Autodesk Inventor part; units mm, degrees
(part 2 of 2)
sketch "Sketch20" plane through (-59.7998, 7.69, 3.5001) normal (0, 0, -1) x (-1, 0, 0)
  line L0 (4.2162, -20.29) -> (4.2162, 0) construction
  line L1 (4.2162, -21.29) -> (44.8074, -21.29) construction
  line L2 (4.2162, 0) -> (4.2162, -21.29) construction
  line L3 (39.8922, -3) -> (33.5483, -3) construction
  line L4 (39.8922, -3) -> (4.2162, -3) construction
  line L5 (4.2162, -3) -> (4.2162, -21.29) construction
  line L6 (4.2162, -21.29) -> (39.8922, -21.29) construction
  line L7 (39.8922, -21.29) -> (39.8922, -3) construction
  line L8 (4.2162, -3) -> (44.8074, -3) construction
  line L9 (44.8074, -3) -> (44.8074, -21.29) construction
  line L10 (44.8074, -21.29) -> (4.2162, -21.29) construction
  line L11 (4.2162, -21.29) -> (4.2162, -3) construction
  line L12 (44.8074, -12.145) -> (4.2162, -12.145) construction
  circle A0 centre (24.5118, -12.145) radius 3.5
  point P0 (-59.7998, -7.69)
  dimension "d266" = 7
  constraints: 22 end point, 4 parallel, 3 horizontal, 3 midpoint, 2 perpendicular, 1 centre point
  measures "d266" diameter of A0
extrude "Extrusion15" cut sketch "Sketch20" along normal blind 100 and the other way blind 50
sketch "Sketch21" plane through (-66.1, 7.69, -7.6) normal (0, 1, 0) x (1, 0, 0)
  line L0 (71.1002, -14.1001) -> (71.1002, 52.1999) projected
  arc A0 (71.1002, 52.1999) -> (67.2926, 61.3923) centre (58.1002, 52.1999) ccw projected
  line L1 (67.2926, 61.3923) -> (47.1426, 81.5423) projected
  arc A1 (47.1426, 81.5423) -> (28.7578, 81.5423) centre (37.9502, 72.3499) ccw projected
  line L2 (28.7578, 81.5423) -> (8.6078, 61.3923) projected
  arc A2 (8.6078, 61.3923) -> (5.0308, 54.6374) centre (17.8002, 52.1999) ccw projected
  arc A3 (2.084, 52.1999) -> (5.0308, 54.6374) centre (2.084, 55.1999) ccw projected
  line L3 (2.084, 52.1999) -> (-68.9958, 52.1999) projected
  arc A4 (-68.9958, 52.1999) -> (-78.1882, 48.3923) centre (-68.9958, 39.1999) ccw projected
  line L4 (-78.1882, 48.3923) -> (-98.3382, 28.2423) projected
  arc A5 (-98.3382, 28.2423) -> (-98.3382, 9.8575) centre (-89.1458, 19.0499) ccw projected
  line L5 (-98.3382, 9.8575) -> (-78.1882, -10.2925) projected
  arc A6 (-78.1882, -10.2925) -> (-68.9958, -14.1001) centre (-68.9958, -1.1001) ccw projected
  line L6 (-68.9958, -14.1001) -> (2.084, -14.1001) projected
  arc A7 (5.0308, -16.5376) -> (2.084, -14.1001) centre (2.084, -17.1001) ccw projected
  arc A8 (5.0308, -16.5376) -> (8.6078, -23.2925) centre (17.8002, -14.1001) ccw projected
  line L7 (8.6078, -23.2925) -> (28.7578, -43.4425) projected
  arc A9 (28.7578, -43.4425) -> (47.1426, -43.4425) centre (37.9502, -34.2501) ccw projected
  line L8 (47.1426, -43.4425) -> (67.2926, -23.2925) projected
  arc A10 (67.2926, -23.2925) -> (71.1002, -14.1001) centre (58.1002, -14.1001) ccw projected
  line L9 (68.1002, 49.1999) -> (68.1002, -10.3919) projected
  line L10 (68.1002, -10.3919) -> (66.5817, -14.6605) projected
  arc A11 (64.1106, -20.1105) -> (66.5817, -14.6605) centre (58.1002, -14.1001) ccw projected
  line L11 (64.1106, -20.1105) -> (43.9606, -40.2605) projected
  arc A12 (31.9398, -40.2605) -> (43.9606, -40.2605) centre (37.9502, -34.2501) ccw projected
  line L12 (31.9398, -40.2605) -> (11.7898, -20.1105) projected
  arc A13 (9.3002, -14.1001) -> (11.7898, -20.1105) centre (17.8002, -14.1001) ccw projected
  arc A14 (9.3002, -14.1001) -> (6.3002, -11.1001) centre (6.3002, -14.1001) ccw projected
  line L13 (6.3002, -11.1001) -> (-38.5071, -11.1001) projected
  arc A15 (-40.6284, -10.2214) -> (-38.5071, -11.1001) centre (-38.5071, -8.1001) ccw projected
  line L14 (-40.6284, -10.2214) -> (-40.3711, -10.4788) projected
  arc A16 (-40.3711, -10.4788) -> (-42.4924, -9.6001) centre (-42.4924, -12.6001) ccw projected
  line L15 (-42.4924, -9.6001) -> (-68.9958, -9.6001) projected
  arc A17 (-75.0062, -7.1105) -> (-68.9958, -9.6001) centre (-68.9958, -1.1001) ccw projected
  line L16 (-75.0062, -7.1105) -> (-95.1562, 13.0395) projected
  arc A18 (-95.1562, 25.0603) -> (-95.1562, 13.0395) centre (-89.1458, 19.0499) ccw projected
  line L17 (-95.1562, 25.0603) -> (-75.0062, 45.2103) projected
  arc A19 (-68.9958, 47.6999) -> (-75.0062, 45.2103) centre (-68.9958, 39.1999) ccw projected
  line L18 (-68.9958, 47.6999) -> (-42.4924, 47.6999) projected
  arc A20 (-42.4924, 47.6999) -> (-40.3711, 48.5786) centre (-42.4924, 50.6999) ccw projected
  line L19 (-40.3711, 48.5786) -> (-40.3356, 48.6141) projected
  arc A21 (-38.9213, 49.1999) -> (-40.3356, 48.6141) centre (-38.9213, 47.1999) ccw projected
  line L20 (-38.9213, 49.1999) -> (6.3002, 49.1999) projected
  arc A22 (6.3002, 49.1999) -> (9.3002, 52.1999) centre (6.3002, 52.1999) ccw projected
  arc A23 (11.7898, 58.2103) -> (9.3002, 52.1999) centre (17.8002, 52.1999) ccw projected
  line L21 (11.7898, 58.2103) -> (31.9398, 78.3603) projected
  arc A24 (43.9606, 78.3603) -> (31.9398, 78.3603) centre (37.9502, 72.3499) ccw projected
  line L22 (43.9606, 78.3603) -> (64.1106, 58.2103) projected
  arc A25 (66.8919, 51.6165) -> (64.1106, 58.2103) centre (57.0713, 51.3576) ccw projected
  line L23 (66.8919, 51.6165) -> (68.1002, 49.1999) projected
  point P0 (66.1, -7.6)
extrude "Extrusion16" add sketch "Sketch21" against normal blind 3 contours A10 L8 A9 L7 A8 A7 L6 A6 L5 A5 L4 A4 L3 A3 A2 L2 A1 L1 A0 L0 | L9 L10 A11 L11 A12 L12 A13 A14 L13 A15 L14 A16 L15 A17 L16 A18 L17 A19 L18 A20 L19 A21 L20 A22 A23 L21 A24 L22 A25 L23
sketch "Sketch22" plane through (-57.4922, -13.6, 15.6925) normal (-0.7071068, 0, 0.7071068) x (0.7071068, 0, 0.7071068)
  line L0 (44.1622, -18.29) -> (71.0798, -18.29) construction
  line L1 (71.0798, -18.29) -> (71.0798, -1) construction
  line L2 (71.0798, -1) -> (44.1622, -1) construction
  line L3 (44.1622, -1) -> (44.1622, -18.29) construction
  line L4 (71.0798, -1) -> (71.0798, -18.29) construction
  line L5 (71.0798, -9.645) -> (44.1622, -9.645) construction
  line L6 (44.1622, -1) -> (44.1622, -18.29) construction
  arc A0 (55.5252, -6.11) -> (61.6635, -6.11) centre (58.5944, -10) ccw
  line L7 (55.5252, -6.11) -> (61.6635, -6.11)
  line L8 (50.344, -9.645) -> (54.4692, -2.5) construction
  line L9 (54.4692, -2.5) -> (62.7195, -2.5) construction
  line L10 (62.7195, -2.5) -> (66.8447, -9.645) construction
  line L11 (66.8447, -9.645) -> (62.7195, -16.79) construction
  line L12 (62.7195, -16.79) -> (54.4692, -16.79) construction
  line L13 (54.4692, -16.79) -> (50.344, -9.645) construction
  line L14 (58.5944, -9.645) -> (54.4692, -2.5) construction
  line L15 (58.5944, -10) -> (58.5944, -1.75) construction
  line L16 (58.5944, -9) -> (66.8444, -9) construction
  line L17 (58.5944, -1) -> (58.5944, -0.8021) construction
  line L18 (58.5944, -9) -> (58.5944, -10) construction
  line L19 (58.5944, -9) -> (59.5944, -9) construction
  line L20 (44.5764, -17.29) -> (44.5764, 3)
  line L21 (71.0798, -17.29) -> (71.0798, 3)
  line L22 (44.5764, 3) -> (71.0798, 3)
  line L23 (71.0798, -17.29) -> (44.5764, -17.29)
  line L24 (0, 0) -> (0, 21.29) projected
  line L25 (28.4964, 0) -> (0, 0) projected
  line L26 (28.4964, 0) -> (28.4964, 21.29) projected
  line L27 (0, 21.29) -> (28.4964, 21.29) projected
  line L28 (24.2613, 8.645) -> (20.1362, 1.5) construction
  line L29 (11.8858, 1.5) -> (7.7607, 8.645) construction
  line L30 (28.4964, 1) -> (1.993, 1)
  line L31 (1.5788, 0) -> (28.4964, 0) construction
  line L32 (28.4964, 8.645) -> (1.5788, 8.645) construction
  line L33 (28.4964, 17.29) -> (28.4964, 0) construction
  line L34 (28.4964, 0) -> (28.4964, 17.29) construction
  line L35 (16.011, 9.29) -> (24.261, 9.29) construction
  line L36 (1.5788, 17.29) -> (1.5788, 0) construction
  line L37 (1.5788, 17.29) -> (1.5788, 0) construction
  line L38 (28.4964, 1) -> (28.4964, 21.29)
  line L39 (1.993, 1) -> (1.993, 21.29)
  line L40 (7.7607, 8.645) -> (11.8858, 15.79) construction
  line L41 (20.1362, 15.79) -> (24.2613, 8.645) construction
  line L42 (11.8858, 15.79) -> (20.1362, 15.79) construction
  line L43 (16.011, 8.29) -> (16.011, 16.54) construction
  line L44 (28.4964, 17.29) -> (1.5788, 17.29) construction
  line L45 (16.011, 17.29) -> (16.011, 17.4879) construction
  line L46 (1.993, 21.29) -> (28.4964, 21.29)
  line L47 (-78.5996, 17.29) -> (28.4964, 17.29) construction
  line L48 (16.011, 9.29) -> (17.011, 9.29) construction
  line L49 (16.011, 9.29) -> (16.011, 8.29) construction
  line L50 (12.9418, 11.831) -> (19.0802, 11.831)
  arc A1 (12.9418, 11.831) -> (19.0802, 11.831) centre (16.011, 7.941) ccw
  line L51 (20.1362, 1.5) -> (11.8858, 1.5) construction
  line L52 (16.011, 8.645) -> (11.8858, 15.79) construction
  line L53 (32.9454, 18.29) -> (29.6309, 18.29) projected
  line L54 (29.6309, 18.29) -> (29.6309, 11.831)
  line L55 (29.6309, 18.29) -> (29.6309, 1) projected
  line L56 (16.011, 12.18) -> (16.011, 11.831)
  point P0 (29.5568, 13.6)
  dimension "d275" = 9.91
  dimension "d276" = 14.29
  dimension "d277" = 8.2503
  dimension "d278" = 8.25
  dimension "d279" = 90
  dimension "d280" = 0.75
  dimension "d281" = 1
  dimension "d282" = 90
  dimension "d283" = 6.1818
  dimension "d284" = 9.91
  dimension "d285" = 14.29
  dimension "d286" = 8.2503
  dimension "d287" = 8.25
  dimension "d288" = 90
  dimension "d289" = 0.75
  dimension "d290" = 1
  dimension "d291" = 90
  dimension "d292" = 6.1818
  dimension "d295" = 6.459
  constraints: 102 end point, 8 horizontal, 7 perpendicular, 6 point on line, 4 midpoint, 4 parallel, 4 point on circle, 2 centre point, 2 vertical, 1 coincident
  measures "d275" diameter of A0
  measures "d276" distance between parallel lines of L9 L12
  measures "d277" distance of L14.start L8.end
  measures "d278" distance of L15.start L15.end
  measures "d279" angle of L16 L15
  measures "d280" distance of L15.end L17.start
  measures "d281" distance of L18.start L18.end
  measures "d282" angle of L18 L19
  measures "d283" distance from line of L3 L13.end
  measures "d284" diameter of A1
  measures "d285" distance between parallel lines of L42 L51
  measures "d286" distance of L52.start L40.end
  measures "d287" distance of L43.start L43.end
  measures "d288" angle of L35 L43
  measures "d289" distance of L43.end L45.start
  measures "d290" distance of L49.start L49.end
  measures "d291" angle of L49 L48
  measures "d292" distance from line of L36 L40.start
  measures "d295" distance of L53.end L54.end
extrude "Extrusion17" cut sketch "Sketch22" against normal blind 5 contours L50 A1
sketch "Sketch23" plane through (-18.9574, -13.6, 35.8425) normal (0.7071068, 0, 0.7071068) x (0.7071068, 0, -0.7071068)
  line L0 (0, 0) -> (0, 21.29) projected
  line L1 (28.4964, 0) -> (0, 0) projected
  line L2 (28.4964, 0) -> (28.4964, 21.29) projected
  line L3 (0, 21.29) -> (28.4964, 21.29) projected
  line L4 (0, 0) -> (0, 21.29)
  line L5 (28.4964, 0) -> (0, 0)
  line L6 (28.4964, 0) -> (28.4964, 21.29)
  line L7 (0, 21.29) -> (28.4964, 21.29)
  line L8 (7.7607, 8.645) -> (11.8858, 15.79) construction
  line L9 (1.993, 1) -> (1.993, 21.29)
  line L10 (16.011, 8.645) -> (11.8858, 15.79) construction
  line L11 (12.9418, 11.831) -> (19.0802, 11.831)
  line L12 (11.8858, 15.79) -> (20.1362, 15.79) construction
  line L13 (11.8858, 1.5) -> (7.7607, 8.645) construction
  arc A0 (12.9418, 11.831) -> (19.0802, 11.831) centre (16.011, 7.941) ccw
  line L14 (20.1362, 1.5) -> (11.8858, 1.5) construction
  line L15 (28.4964, 17.29) -> (1.5788, 17.29) construction
  line L16 (28.4964, 8.645) -> (1.5788, 8.645) construction
  line L17 (28.4964, 1) -> (1.993, 1)
  line L18 (28.4964, 17.29) -> (28.4964, 0) construction
  line L19 (28.4964, 0) -> (28.4964, 17.29) construction
  line L20 (1.5788, 0) -> (28.4964, 0) construction
  line L21 (1.5788, 17.29) -> (1.5788, 0) construction
  line L22 (1.5788, 17.29) -> (1.5788, 0) construction
  line L23 (24.2613, 8.645) -> (20.1362, 1.5) construction
  line L24 (16.011, 17.29) -> (16.011, 17.4879) construction
  line L25 (16.011, 8.29) -> (16.011, 16.54) construction
  line L26 (16.011, 9.29) -> (16.011, 8.29) construction
  line L27 (16.011, 9.29) -> (17.011, 9.29) construction
  line L28 (16.011, 9.29) -> (24.261, 9.29) construction
  line L29 (28.4964, 1) -> (28.4964, 21.29)
  line L30 (20.1362, 15.79) -> (24.2613, 8.645) construction
  line L31 (-78.5996, 17.29) -> (28.4964, 17.29) construction
  line L32 (1.993, 21.29) -> (28.4964, 21.29)
  line L33 (32.9454, 18.29) -> (29.6309, 18.29)
  line L34 (29.6309, 18.29) -> (29.6309, 11.831)
  line L35 (29.6309, 18.29) -> (29.6309, 1)
  line L36 (16.011, 12.18) -> (16.011, 11.831)
  point P0 (38.7494, 13.6)
  point P1 (29.5568, 13.6)
  dimension "d297" = 9.91
  dimension "d298" = 14.29
  dimension "d299" = 8.2503
  dimension "d300" = 8.25
  dimension "d301" = 90
  dimension "d302" = 0.75
  dimension "d303" = 1
  dimension "d304" = 90
  dimension "d305" = 6.1818
  dimension "d306" = 6.459
  constraints: 66 end point, 5 point on line, 4 horizontal, 4 perpendicular, 2 midpoint, 2 parallel, 2 point on circle, 1 centre point, 1 vertical
  measures "d297" diameter of A0
  measures "d298" distance between parallel lines of L12 L14
  measures "d299" distance of L10.start L8.end
  measures "d300" distance of L25.start L25.end
  measures "d301" angle of L28 L25
  measures "d302" distance of L25.end L24.start
  measures "d303" distance of L26.start L26.end
  measures "d304" angle of L26 L27
  measures "d305" distance from line of L21 L13.end
  measures "d306" distance of L35.start L34.end
extrude "Extrusion18" cut sketch "Sketch23" against normal blind 5 contours L11 A0
sketch "Sketch24" plane through (1.1926, -13.6, -68.9923) normal (0.7071068, 0, -0.7071068) x (-0.7071068, 0, -0.7071068)
  line L0 (0, 0) -> (0, 21.29) projected
  line L1 (28.4964, 0) -> (0, 0) projected
  line L2 (28.4964, 0) -> (28.4964, 21.29) projected
  line L3 (0, 21.29) -> (28.4964, 21.29) projected
  line L4 (0, 0) -> (0, 21.29)
  line L5 (28.4964, 0) -> (0, 0)
  line L6 (28.4964, 0) -> (28.4964, 21.29)
  line L7 (0, 21.29) -> (28.4964, 21.29)
  line L8 (7.7607, 8.645) -> (11.8858, 15.79) construction
  line L9 (1.993, 1) -> (1.993, 21.29)
  line L10 (16.011, 8.645) -> (11.8858, 15.79) construction
  line L11 (12.9418, 11.831) -> (19.0802, 11.831)
  line L12 (11.8858, 15.79) -> (20.1362, 15.79) construction
  line L13 (11.8858, 1.5) -> (7.7607, 8.645) construction
  arc A0 (12.9418, 11.831) -> (19.0802, 11.831) centre (16.011, 7.941) ccw
  line L14 (20.1362, 1.5) -> (11.8858, 1.5) construction
  line L15 (28.4964, 17.29) -> (1.5788, 17.29) construction
  line L16 (28.4964, 8.645) -> (1.5788, 8.645) construction
  line L17 (28.4964, 1) -> (1.993, 1)
  line L18 (28.4964, 17.29) -> (28.4964, 0) construction
  line L19 (28.4964, 0) -> (28.4964, 17.29) construction
  line L20 (1.5788, 0) -> (28.4964, 0) construction
  line L21 (1.5788, 17.29) -> (1.5788, 0) construction
  line L22 (1.5788, 17.29) -> (1.5788, 0) construction
  line L23 (24.2613, 8.645) -> (20.1362, 1.5) construction
  line L24 (16.011, 17.29) -> (16.011, 17.4879) construction
  line L25 (16.011, 8.29) -> (16.011, 16.54) construction
  line L26 (16.011, 9.29) -> (16.011, 8.29) construction
  line L27 (16.011, 9.29) -> (17.011, 9.29) construction
  line L28 (16.011, 9.29) -> (24.261, 9.29) construction
  line L29 (28.4964, 1) -> (28.4964, 21.29)
  line L30 (20.1362, 15.79) -> (24.2613, 8.645) construction
  line L31 (-78.5996, 17.29) -> (28.4964, 17.29) construction
  line L32 (1.993, 21.29) -> (28.4964, 21.29)
  line L33 (32.9454, 18.29) -> (29.6309, 18.29)
  line L34 (29.6309, 18.29) -> (29.6309, 11.831)
  line L35 (29.6309, 18.29) -> (29.6309, 1)
  line L36 (16.011, 12.18) -> (16.011, 11.831)
  line L37 (29.6309, 18.29) -> (16.011, 18.29)
  line L38 (23.5519, 18.29) -> (-8.1317, 18.29) projected
  line L39 (16.011, 18.29) -> (16.011, 12.18)
  line L40 (16.011, 30.1424) -> (15.662, 30.1424)
  point P0 (-47.9416, 13.6)
  point P1 (29.5568, 13.6)
  dimension "d309" = 9.91
  dimension "d310" = 14.29
  dimension "d311" = 8.2503
  dimension "d312" = 8.25
  dimension "d313" = 90
  dimension "d314" = 0.75
  dimension "d315" = 1
  dimension "d316" = 90
  dimension "d317" = 6.1818
  dimension "d318" = 6.459
  dimension "d339" = 4
  dimension "d340" = 3
  dimension "d341" = 6.11
  dimension "d342" = 0.349
  constraints: 72 end point, 6 point on line, 5 horizontal, 4 perpendicular, 2 midpoint, 2 parallel, 2 point on circle, 1 centre point, 1 collinear, 1 vertical
  measures "d309" diameter of A0
  measures "d310" distance between parallel lines of L12 L14
  measures "d311" distance of L10.start L10.end
  measures "d312" distance of L25.start L25.end
  measures "d313" angle of L28 L25
  measures "d314" distance of L25.end L24.start
  measures "d315" distance of L26.start L26.end
  measures "d316" angle of L26 L27
  measures "d317" distance from line of L21 L8.start
  measures "d318" distance of L34.start L34.end
  measures "d339" distance between parallel lines of L3 L15
  measures "d340" distance between parallel lines of L33 L7
  measures "d341" distance of L37.end L36.start
  measures "d342" distance of L40.start L40.end
sketch "Sketch25" plane through (-37.3422, -13.6, -89.1423) normal (-0.7071068, 0, -0.7071068) x (-0.7071068, 0, 0.7071068)
  line L0 (0, 0) -> (0, 21.29) projected
  line L1 (28.4964, 0) -> (0, 0) projected
  line L2 (28.4964, 0) -> (28.4964, 21.29) projected
  line L3 (0, 21.29) -> (28.4964, 21.29) projected
  line L4 (0, 0) -> (0, 21.29)
  line L5 (28.4964, 0) -> (0, 0)
  line L6 (28.4964, 0) -> (28.4964, 21.29)
  line L7 (0, 21.29) -> (28.4964, 21.29)
  line L8 (7.7607, 8.645) -> (11.8858, 15.79) construction
  line L9 (1.993, 1) -> (1.993, 21.29)
  line L10 (16.011, 8.645) -> (11.8858, 15.79) construction
  line L11 (12.9418, 11.831) -> (19.0802, 11.831)
  line L12 (11.8858, 15.79) -> (20.1362, 15.79) construction
  line L13 (11.8858, 1.5) -> (7.7607, 8.645) construction
  arc A0 (12.9418, 11.831) -> (19.0802, 11.831) centre (16.011, 7.941) ccw
  line L14 (20.1362, 1.5) -> (11.8858, 1.5) construction
  line L15 (28.4964, 17.29) -> (1.5788, 17.29) construction
  line L16 (28.4964, 8.645) -> (1.5788, 8.645) construction
  line L17 (28.4964, 1) -> (1.993, 1)
  line L18 (28.4964, 17.29) -> (28.4964, 0) construction
  line L19 (28.4964, 0) -> (28.4964, 17.29) construction
  line L20 (1.5788, 0) -> (28.4964, 0) construction
  line L21 (1.5788, 17.29) -> (1.5788, 0) construction
  line L22 (1.5788, 17.29) -> (1.5788, 0) construction
  line L23 (24.2613, 8.645) -> (20.1362, 1.5) construction
  line L24 (16.011, 17.29) -> (16.011, 17.4879) construction
  line L25 (16.011, 8.29) -> (16.011, 16.54) construction
  line L26 (16.011, 9.29) -> (16.011, 8.29) construction
  line L27 (16.011, 9.29) -> (17.011, 9.29) construction
  line L28 (16.011, 9.29) -> (24.261, 9.29) construction
  line L29 (28.4964, 1) -> (28.4964, 21.29)
  line L30 (20.1362, 15.79) -> (24.2613, 8.645) construction
  line L31 (-78.5996, 17.29) -> (28.4964, 17.29) construction
  line L32 (1.993, 21.29) -> (28.4964, 21.29)
  line L33 (32.9454, 18.29) -> (29.6309, 18.29)
  line L34 (29.6309, 18.29) -> (29.6309, 11.831)
  line L35 (29.6309, 18.29) -> (29.6309, 1)
  line L36 (16.011, 12.18) -> (16.011, 11.831)
  point P0 (36.6282, 13.6)
  point P1 (29.5568, 13.6)
  dimension "d319" = 9.91
  dimension "d320" = 14.29
  dimension "d321" = 8.2503
  dimension "d322" = 8.25
  dimension "d323" = 90
  dimension "d324" = 0.75
  dimension "d325" = 1
  dimension "d326" = 90
  dimension "d327" = 6.1818
  dimension "d328" = 6.459
  constraints: 66 end point, 5 point on line, 4 horizontal, 4 perpendicular, 2 midpoint, 2 parallel, 2 point on circle, 1 centre point, 1 vertical
  measures "d319" diameter of A0
  measures "d320" distance between parallel lines of L12 L14
  measures "d321" distance of L10.start L10.end
  measures "d322" distance of L25.start L25.end
  measures "d323" angle of L28 L25
  measures "d324" distance of L25.end L24.start
  measures "d325" distance of L26.start L26.end
  measures "d326" angle of L26 L27
  measures "d327" distance from line of L21 L8.start
  measures "d328" distance of L34.start L34.end
extrude "Extrusion19" cut sketch "Sketch25" against normal blind 5 contours L11 A0
extrude "Extrusion20" cut sketch "Sketch24" against normal blind 5 contours L11 A0
sketch "Sketch27" plane through (-66.1, 4.69, -7.6) normal (0, -1, 0) x (1, 0, 0)
  line L0 (68.1002, 5.7045) -> (71.1002, 5.7045) projected
  line L1 (71.1002, -6.0043) -> (68.1002, -6.0043) projected
  line L2 (68.1002, 5.7045) -> (71.1002, 5.7045)
  line L3 (71.1002, 5.7045) -> (71.1002, -6.0043)
  line L4 (71.1002, -6.0043) -> (68.1002, -6.0043)
  line L5 (68.1002, -6.0043) -> (68.1002, 5.7045)
  line L6 (71.1002, -37.9894) -> (71.1002, -21.9894) projected
  line L7 (71.1002, -37.9894) -> (68.1002, -37.9894) projected
  line L8 (71.1002, -21.9894) -> (68.1002, -21.9894)
  line L9 (68.1002, -21.9894) -> (68.1002, -37.9894)
  line L10 (68.1002, -37.9894) -> (71.1002, -37.9894)
  line L11 (71.1002, -37.9894) -> (71.1002, -21.9894)
  point P0 (66.1, 7.6)
  constraints: 16 end point, 4 parallel, 2 horizontal, 2 perpendicular
extrude "Extrusion21" add sketch "Sketch27" along normal blind 6.29
body "Solid1"
